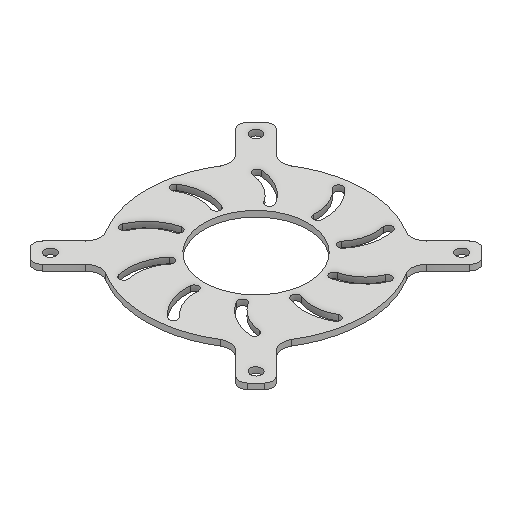
# Autodesk Inventor part: 3DP_ABS_Chamber_Fan_Cover
Saved by Autodesk Inventor 2026.1 (Build 301233000, 233)
## iProperties
Created: 2017-07-28
Part Number: 3DP_ABS_Chamber_Fan_Cover
Material: Ogólny
Document SubType Name: Modeling
Designer: Andrzej
Density: 1 g/cm^3
Appearance: Default
Author: Andrzej
Autodesk Inventor part; units mm, degrees
ref_plane "YZ Plane" through (0, 0, 0) normal (1, 0, 0) x (0, 1, 0)
ref_plane "XZ Plane" through (0, 0, 0) normal (0, 1, 0) x (-1, 0, 0)
ref_plane "XY Plane" through (0, 0, 0) normal (0, 0, 1) x (1, 0, 0)
sketch "Szkic1" plane through (0, 0, 0) normal (0, 0, 1) x (1, 0, 0)
  circle A0 centre (-27.3367, -1.5929) radius 18
  circle A1 centre (-27.3367, -1.5929) radius 38
  line L0 (-63.0867, 41.2281) -> (-70.1578, 34.1571)
  line L1 (8.4133, 41.2281) -> (15.4843, 34.1571)
  line L2 (-70.1578, -37.3429) -> (-63.0867, -44.414)
  line L3 (8.4133, -44.414) -> (15.4843, -37.3429)
  line L4 (-70.1578, 34.1571) -> (-57.5087, 21.508)
  line L5 (-70.1578, -37.3429) -> (-57.5087, -24.6938)
  line L6 (-63.0867, 41.2281) -> (-50.4376, 28.579)
  line L7 (-4.2358, 28.579) -> (8.4133, 41.2281)
  line L8 (2.8352, 21.508) -> (15.4843, 34.1571)
  line L9 (2.8352, -24.6938) -> (15.4843, -37.3429)
  line L10 (-4.2358, -31.7649) -> (8.4133, -44.414)
  line L11 (-63.0867, -44.414) -> (-50.4376, -31.7649)
  point P0 (0, 0)
  point P1 (-63.0867, 34.1571)
  point P2 (8.4133, 34.1571)
  point P3 (-63.0867, -37.3429)
  point P4 (8.4133, -37.3429)
  dimension "d5" = 76
  dimension "d0" = 71.5
  dimension "d1" = 71.5
  dimension "d2" = 35.75
  dimension "d3" = 35.75
  dimension "d4" = 36
  dimension "d14" = 5
  dimension "d15" = 5
  dimension "d16" = 5
  dimension "d17" = 5
  constraints: 24 end point, 8 parallel, 8 perpendicular, 2 coincident, 2 horizontal alignment, 2 vertical alignment, 1 centre point, 10 other
  measures "d0" distance of point (-63.087, 34.157) point (-63.087, -37.343)
  measures "d1" distance of point (8.413, -37.343) point (-63.087, -37.343)
  measures "d2" horizontal distance of point (-63.087, 34.157) point (-27.337, -1.593)
  measures "d3" horizontal distance of point (-63.087, -37.343) point (-27.337, -1.593)
  measures "d4" diameter of A0
  measures "d14" distance from line of L2 point (-63.087, -37.343)
  measures "d15" distance from line of L0 point (-63.087, 34.157)
  measures "d16" distance from line of L1 point (8.413, 34.157)
  measures "d17" distance from line of point (8.413, -37.343) L3
extrude "Wyciągnięcie proste1" add sketch "Szkic1" along normal blind 2
hole "Otwór1" at (-63.0867, 34.1571, 0) at (8.4133, 34.1571, 0) at (-63.0867, -37.3429, 0) at (8.4133, -37.3429, 0) at (-27.3367, -1.5929, 0) direction (0, 0, 1) diameter 4 end through all
fillet "Zaokrąglenie1" radius 3 8 edges at (-63.0867, 41.2281, 1) (15.4843, 34.1571, 1) (8.4133, 41.2281, 1) (-70.1578, 34.1571, 1) (-63.0867, -44.414, 1) (-70.1578, -37.3429, 1) (15.4843, -37.3429, 1) (8.4133, -44.414, 1)
fillet "Zaokrąglenie1" radius 5 8 edges at (-57.5087, 21.508, 1) (-50.4376, 28.579, 1) (-57.5087, -24.6938, 1) (-50.4376, -31.7649, 1) (-4.2358, -31.7649, 1) (2.8352, -24.6938, 1) (-4.2358, 28.579, 1) (2.8352, 21.508, 1)
sketch "Szkic2" plane through (0, 0, 2) normal (0, 0, 1) x (1, 0, 0)
  circle A0 centre (8.4133, -37.3429) radius 2 projected
  circle A1 centre (8.4133, 34.1571) radius 2 projected
  circle A2 centre (-63.0867, 34.1571) radius 2 projected
  circle A3 centre (-63.0867, -37.3429) radius 2 projected
  circle A4 centre (-27.3367, -1.5929) radius 18 projected
  arc A5 (6.2919, -42.2927) -> (10.5346, -42.2927) centre (8.4133, -40.1714) ccw projected
  line L0 (10.5346, -42.2927) -> (13.363, -39.4643) projected
  arc A6 (13.363, -39.4643) -> (13.363, -35.2216) centre (11.2417, -37.3429) ccw projected
  line L1 (13.363, -35.2216) -> (5.7707, -27.6293) projected
  arc A7 (5.0455, -21.4774) -> (5.7707, -27.6293) centre (9.3063, -24.0938) ccw projected
  arc A8 (5.0455, -21.4774) -> (5.0455, 18.2916) centre (-27.3367, -1.5929) ccw projected
  arc A9 (5.7707, 24.4435) -> (5.0455, 18.2916) centre (9.3063, 20.9079) ccw projected
  line L2 (5.7707, 24.4435) -> (13.363, 32.0357) projected
  arc A10 (13.363, 32.0357) -> (13.363, 36.2784) centre (11.2417, 34.1571) ccw projected
  line L3 (13.363, 36.2784) -> (10.5346, 39.1068) projected
  arc A11 (10.5346, 39.1068) -> (6.2919, 39.1068) centre (8.4133, 36.9855) ccw projected
  line L4 (6.2919, 39.1068) -> (-1.3003, 31.5145) projected
  arc A12 (-7.4522, 30.7893) -> (-1.3003, 31.5145) centre (-4.8359, 35.0501) ccw projected
  arc A13 (-7.4522, 30.7893) -> (-47.2212, 30.7893) centre (-27.3367, -1.5929) ccw projected
  arc A14 (-53.3731, 31.5145) -> (-47.2212, 30.7893) centre (-49.8376, 35.0501) ccw projected
  line L5 (-53.3731, 31.5145) -> (-60.9654, 39.1068) projected
  arc A15 (-60.9654, 39.1068) -> (-65.2081, 39.1068) centre (-63.0867, 36.9855) ccw projected
  line L6 (-65.2081, 39.1068) -> (-68.0365, 36.2784) projected
  arc A16 (-68.0365, 36.2784) -> (-68.0365, 32.0357) centre (-65.9152, 34.1571) ccw projected
  line L7 (-68.0365, 32.0357) -> (-60.4442, 24.4435) projected
  arc A17 (-59.7189, 18.2916) -> (-60.4442, 24.4435) centre (-63.9797, 20.9079) ccw projected
  arc A18 (-59.7189, 18.2916) -> (-59.7189, -21.4774) centre (-27.3367, -1.5929) ccw projected
  arc A19 (-60.4442, -27.6293) -> (-59.7189, -21.4774) centre (-63.9797, -24.0938) ccw projected
  line L8 (-60.4442, -27.6293) -> (-68.0365, -35.2216) projected
  arc A20 (-68.0365, -35.2216) -> (-68.0365, -39.4643) centre (-65.9152, -37.3429) ccw projected
  line L9 (-68.0365, -39.4643) -> (-65.2081, -42.2927) projected
  arc A21 (-65.2081, -42.2927) -> (-60.9654, -42.2927) centre (-63.0867, -40.1714) ccw projected
  line L10 (-60.9654, -42.2927) -> (-53.3731, -34.7004) projected
  arc A22 (-47.2212, -33.9751) -> (-53.3731, -34.7004) centre (-49.8376, -38.2359) ccw projected
  arc A23 (-47.2212, -33.9751) -> (-7.4522, -33.9751) centre (-27.3367, -1.5929) ccw projected
  arc A24 (-1.3003, -34.7004) -> (-7.4522, -33.9751) centre (-4.8359, -38.2359) ccw projected
  line L11 (-1.3003, -34.7004) -> (6.2919, -42.2927) projected
  line L12 (-27.3367, 32.9071) -> (-27.3367, 19.9071)
  arc A25 (-27.3367, 19.9071) -> (-32.3762, 32.1571) centre (-42.2339, 20.9402) ccw construction
  arc A26 (-25.8403, 19.8033) -> (-31.386, 33.2838) centre (-42.2339, 20.9402) ccw
  arc A27 (-28.8331, 20.0108) -> (-33.3664, 31.0303) centre (-42.2339, 20.9402) ccw
  arc A28 (-28.8331, 20.0108) -> (-25.8403, 19.8033) centre (-27.3367, 19.9071) ccw
  arc A29 (-31.386, 33.2838) -> (-33.3664, 31.0303) centre (-32.3762, 32.1571) ccw
  arc A30 (-41.2457, 15.0053) -> (-38.7025, 16.5965) centre (-39.9741, 15.8009) ccw
  arc A31 (-38.7025, 16.5965) -> (-51.1127, 24.2428) centre (-52.6334, 7.8804) ccw
  arc A32 (-39.9741, 15.8009) -> (-51.2515, 22.7493) centre (-52.6334, 7.8804) ccw construction
  arc A33 (-41.2457, 15.0053) -> (-51.3903, 21.2557) centre (-52.6334, 7.8804) ccw
  arc A34 (-51.1127, 24.2428) -> (-51.3903, 21.2557) centre (-51.2515, 22.7493) ccw
  arc A35 (-48.3456, 3.6598) -> (-47.2233, 6.442) centre (-47.7844, 5.0509) ccw
  arc A36 (-47.2233, 6.442) -> (-61.7578, 5.3335) centre (-53.3705, -8.7979) ccw
  arc A37 (-47.7844, 5.0509) -> (-60.9922, 4.0436) centre (-53.3705, -8.7979) ccw construction
  arc A38 (-48.3456, 3.6598) -> (-60.2266, 2.7536) centre (-53.3705, -8.7979) ccw
  arc A39 (-61.7578, 5.3335) -> (-60.2266, 2.7536) centre (-60.9922, 4.0436) ccw
  arc A40 (-47.4207, -9.692) -> (-48.1482, -6.7816) centre (-47.7844, -8.2368) ccw
  arc A41 (-48.1482, -6.7816) -> (-59.2552, -16.2215) centre (-44.1635, -22.7241) ccw
  arc A42 (-47.7844, -8.2368) -> (-57.8776, -16.8151) centre (-44.1635, -22.7241) ccw construction
  arc A43 (-47.4207, -9.692) -> (-56.5, -17.4086) centre (-44.1635, -22.7241) ccw
  arc A44 (-59.2552, -16.2215) -> (-56.5, -17.4086) centre (-57.8776, -16.8151) ccw
  arc A45 (-38.8245, -19.9503) -> (-41.1237, -18.0233) centre (-39.9741, -18.9868) ccw
  arc A46 (-41.1237, -18.0233) -> (-44.5608, -32.1889) centre (-28.5293, -28.5789) ccw
  arc A47 (-39.9741, -18.9868) -> (-43.0975, -31.8594) centre (-28.5293, -28.5789) ccw construction
  arc A48 (-38.8245, -19.9503) -> (-41.6341, -31.5299) centre (-28.5293, -28.5789) ccw
  arc A49 (-44.5608, -32.1889) -> (-41.6341, -31.5299) centre (-43.0975, -31.8594) ccw
  arc A50 (-25.8403, -23.1967) -> (-28.8331, -22.9892) centre (-27.3367, -23.0929) ccw
  arc A51 (-28.8331, -22.9892) -> (-23.2874, -36.4697) centre (-12.4395, -24.126) ccw
  arc A52 (-27.3367, -23.0929) -> (-22.2973, -35.3429) centre (-12.4395, -24.126) ccw construction
  arc A53 (-25.8403, -23.1967) -> (-21.3071, -34.2162) centre (-12.4395, -24.126) ccw
  arc A54 (-23.2874, -36.4697) -> (-21.3071, -34.2162) centre (-22.2973, -35.3429) ccw
  arc A55 (-13.4277, -18.1912) -> (-15.971, -19.7824) centre (-14.6993, -18.9868) ccw
  arc A56 (-15.971, -19.7824) -> (-3.5608, -27.4287) centre (-2.04, -11.0662) ccw
  arc A57 (-14.6993, -18.9868) -> (-3.422, -25.9351) centre (-2.04, -11.0662) ccw construction
  arc A58 (-13.4277, -18.1912) -> (-3.2831, -24.4416) centre (-2.04, -11.0662) ccw
  arc A59 (-3.5608, -27.4287) -> (-3.2831, -24.4416) centre (-3.422, -25.9351) ccw
  arc A60 (-6.3279, -6.8457) -> (-7.4501, -9.6279) centre (-6.889, -8.2368) ccw
  arc A61 (-7.4501, -9.6279) -> (7.0843, -8.5193) centre (-1.303, 5.612) ccw
  arc A62 (-6.889, -8.2368) -> (6.3187, -7.2294) centre (-1.303, 5.612) ccw construction
  arc A63 (-6.3279, -6.8457) -> (5.5531, -5.9395) centre (-1.303, 5.612) ccw
  arc A64 (7.0843, -8.5193) -> (5.5531, -5.9395) centre (6.3187, -7.2294) ccw
  arc A65 (-7.2527, 6.5062) -> (-6.5253, 3.5957) centre (-6.889, 5.0509) ccw
  arc A66 (-6.5253, 3.5957) -> (4.5817, 13.0357) centre (-10.51, 19.5382) ccw
  arc A67 (-6.889, 5.0509) -> (3.2041, 13.6292) centre (-10.51, 19.5382) ccw construction
  arc A68 (-7.2527, 6.5062) -> (1.8266, 14.2228) centre (-10.51, 19.5382) ccw
  arc A69 (4.5817, 13.0357) -> (1.8266, 14.2228) centre (3.2041, 13.6292) ccw
  arc A70 (-15.849, 16.7644) -> (-13.5497, 14.8374) centre (-14.6993, 15.8009) ccw
  arc A71 (-13.5497, 14.8374) -> (-10.1126, 29.003) centre (-26.1442, 25.3931) ccw
  arc A72 (-14.6993, 15.8009) -> (-11.576, 28.6735) centre (-26.1442, 25.3931) ccw construction
  arc A73 (-15.849, 16.7644) -> (-13.0394, 28.344) centre (-26.1442, 25.3931) ccw
  arc A74 (-10.1126, 29.003) -> (-13.0394, 28.344) centre (-11.576, 28.6735) ccw
  point P0 (0, 0)
  dimension "d29" = 13
  dimension "d30" = 21.5
  dimension "d31" = 3
  dimension "d34" = 360
  constraints: 100 point on circle, 50 centre point, 4 tangent, 2 end point, 1 vertical, 121 other
  measures "d29" distance of L12.start L12.end
  measures "d30" distance of A4.centre L12.end
  measures "d31" diameter of A29
extrude "Wyciągnięcie proste2" cut sketch "Szkic2" against normal through all contours A28 A27 A29 A26 | A33 A34 A31 A30 | A38 A39 A36 A35 | A43 A44 A41 A40 | A48 A49 A46 A45 | A53 A54 A51 A50 | A58 A59 A56 A55 | A63 A64 A61 A60 | A68 A69 A66 A65 | A73 A74 A71 A70
equation "\"d1\" = d0"
equation "\"d2\" = 0.5 * d0"
equation "\"d3\" = 0.5 * d1"
equation "\"d11\" = d10"
equation "\"d12\" = d10"
equation "\"d13\" = d12"
equation "\"d10\" = 5"
